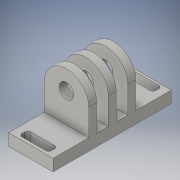
# Autodesk Inventor part: gopro_drone
Saved by Autodesk Inventor 2016 (Build 200138000, 138)
## iProperties
Created: 2015-08-22
Part Number: gopro_drone
Material: Generic
Document SubType Name: Modeling
Designer: Tyler
Density: 1 g/cm^3
Appearance: Default
Author: Tyler
Autodesk Inventor part; units mm, degrees
ref_plane "YZ Plane" through (0, 0, 0) normal (1, 0, 0) x (0, 1, 0)
ref_plane "XZ Plane" through (0, 0, 0) normal (0, 1, 0) x (-1, 0, 0)
ref_plane "XY Plane" through (0, 0, 0) normal (0, 0, 1) x (1, 0, 0)
sketch "Sketch4" plane through (0, 0, 0) normal (0, 0, 1) x (1, 0, 0)
  line L0 (-10.5, 0) -> (10.5, 0) projected
  line L1 (0, -3.3) -> (0, 19.8) projected
  line L2 (-7.5, 0) -> (7.5, 0)
  line L3 (7.5, 0) -> (7.5, 16.5)
  line L4 (7.5, 16.5) -> (-7.5, 16.5)
  line L5 (-7.5, 16.5) -> (-7.5, 0)
  circle A0 centre (0, 10) radius 2.5
  point P0 (0, 0)
  dimension "d0" = 7.5
  dimension "d1" = 7.5
  dimension "d2" = 16.5
  dimension "d3" = 5
  dimension "d4" = 6.5
  constraints: 8 end point, 2 parallel, 2 point on line, 1 centre point, 1 horizontal, 1 perpendicular
  measures "d0" distance between parallel lines of L1 L5
  measures "d1" distance between parallel lines of L1 L3
  measures "d2" distance between parallel lines of L4 L0
  measures "d3" diameter of A0
  measures "d4" distance from line of L4 A0.centre
extrude "Extrusion1" add sketch "Sketch4" against normal blind 15.9 contours L5 L4 L1 A0 L0 | L1 A0 L4 L3 L0
fillet "Fillet1" radius 7.5 2 edges at (7.5, 16.5, -7.95) (-7.5, 16.5, -7.95)
sketch "Sketch10" plane through (-7.5, 0, 0) normal (0, -1, 0) x (1, 0, 0)
  line L0 (-3, 0) -> (18, 0) projected
  line L1 (7.5, -19.08) -> (7.5, 3.18) projected
  line L2 (15, 12.05) -> (0, 12.05)
  line L3 (0, 12.05) -> (0, -27.95)
  line L4 (0, -27.95) -> (15, -27.95)
  line L5 (15, -27.95) -> (15, 12.05)
  line L6 (11.5, 11.05) -> (3.5, 11.05)
  line L7 (2.5, 10.05) -> (2.5, 9.05)
  line L8 (3.5, 8.05) -> (11.5, 8.05)
  line L9 (12.5, 9.05) -> (12.5, 10.05)
  line L10 (15, 0) -> (15, -15.9) projected
  line L11 (15, -8.075) -> (0, -8.075)
  line L12 (0, -15.9) -> (0, 0) projected
  line L13 (11.5, -27.2) -> (3.5, -27.2)
  line L14 (2.5, -26.2) -> (2.5, -25.2)
  line L15 (3.5, -24.2) -> (11.5, -24.2)
  line L16 (12.5, -25.2) -> (12.5, -26.2)
  arc A0 (11.5, 8.05) -> (12.5, 9.05) centre (11.5, 9.05) ccw
  arc A1 (12.5, 10.05) -> (11.5, 11.05) centre (11.5, 10.05) ccw
  arc A2 (3.5, 11.05) -> (2.5, 10.05) centre (3.5, 10.05) ccw
  arc A3 (2.5, 9.05) -> (3.5, 8.05) centre (3.5, 9.05) ccw
  arc A4 (12.5, -25.2) -> (11.5, -24.2) centre (11.5, -25.2) ccw
  arc A5 (11.5, -27.2) -> (12.5, -26.2) centre (11.5, -26.2) ccw
  arc A6 (3.5, -24.2) -> (2.5, -25.2) centre (3.5, -25.2) ccw
  arc A7 (2.5, -26.2) -> (3.5, -27.2) centre (3.5, -26.2) ccw
  point P0 (7.5, 0)
  point P1 (12.5, 11.05)
  point P2 (2.5, 8.05)
  point P3 (2.5, 11.05)
  point P4 (12.5, 8.05)
  point P5 (15, -6.55)
  point P6 (15, -9.6)
  point P7 (0, -9.6)
  point P8 (0, -6.55)
  point P9 (12.5, -27.2)
  point P10 (2.5, -24.2)
  point P11 (2.5, -27.2)
  point P12 (12.5, -24.2)
  point P13 (15, -2.8)
  dimension "d20" = 15
  dimension "d21" = 40
  dimension "d22" = 12.05
  dimension "d23" = 7.5
  dimension "d24" = 3
  dimension "d25" = 1
  dimension "d26" = 10
  dimension "d27" = 2.5
  dimension "d28" = 8.075
  dimension "d29" = 1
  constraints: 26 end point, 18 point on line, 16 point on circle, 16 tangent, 8 centre point, 7 equal radius, 4 parallel, 4 symmetric about line, 2 horizontal, 2 perpendicular
  measures "d20" distance of L2.start L2.end
  measures "d21" distance between parallel lines of L4 L2
  measures "d22" distance between parallel lines of L0 L2
  measures "d23" distance between parallel lines of L1 L5
  measures "d24" distance between parallel lines of L8 L6
  measures "d25" distance between parallel lines of L6 L2
  measures "d26" distance between parallel lines of L7 L9
  measures "d27" distance between parallel lines of L5 L9
  measures "d28" distance between parallel lines of L0 L11
  measures "d29" radius of A0
extrude "Extrusion5" add sketch "Sketch10" along normal blind 4
sketch "Sketch13" plane through (7.5, 9, 0) normal (1, 0, 0) x (0, 0, -1)
  line L0 (0, -17.1) -> (0, 11.6) projected
  line L1 (35.95, -9) -> (-20.05, -9) projected
  line L2 (0, -9) -> (0, 0) projected
  line L3 (0, 7.5) -> (15.9, 7.5) projected
  line L4 (0, -9) -> (2.7, -9)
  line L5 (2.7, -9) -> (2.7, 7.5)
  line L6 (2.7, 7.5) -> (0, 7.5)
  line L7 (0, 7.5) -> (0, -9)
  line L8 (15.9, -9) -> (15.9, 0) projected
  line L9 (15.9, -9) -> (13.2, -9)
  line L10 (13.2, -9) -> (13.2, 7.5)
  line L11 (13.2, 7.5) -> (15.9, 7.5)
  line L12 (15.9, 7.5) -> (15.9, -9)
  line L13 (6.6, -9) -> (9.3, -9)
  line L14 (9.3, -9) -> (9.3, 7.5)
  line L15 (9.3, 7.5) -> (6.6, 7.5)
  line L16 (6.6, 7.5) -> (6.6, -9)
  dimension "d47" = 2.7
  dimension "d48" = 2.7
  dimension "d49" = 2.7
  dimension "d50" = 15.9
  dimension "d51" = 3.9
  dimension "d52" = 3.9
  constraints: 24 end point, 6 parallel, 4 point on line, 3 horizontal, 3 perpendicular
  measures "d47" distance between parallel lines of L5 L0
  measures "d48" distance between parallel lines of L12 L10
  measures "d49" distance between parallel lines of L14 L16
  measures "d50" distance between parallel lines of L12 L0
  measures "d51" distance between parallel lines of L16 L5
  measures "d52" distance between parallel lines of L10 L14
extrude "Extrusion8" cut sketch "Sketch13" against normal through all contours L5 L3 L16 L1 | L14 L3 L10 L1
body "Solid1"
